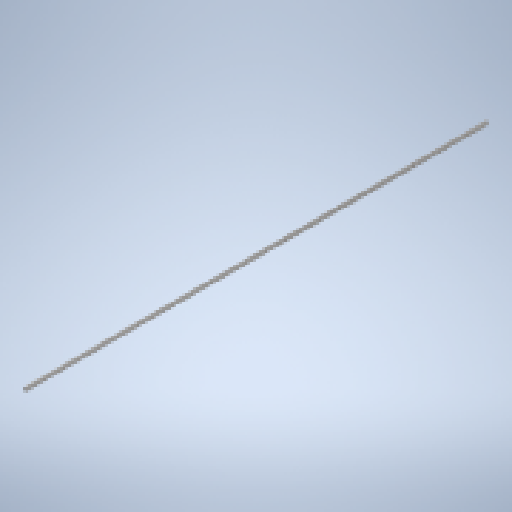
# Autodesk Inventor part: Guia Linear 490mm
Saved by Autodesk Inventor 2025.1 (Build 291241000, 241)
## iProperties
Created: 2020-11-03
Part Number: Guia Linear 490mm
Material: Aço, carbono
Document SubType Name: Modeling
Designer: Mateus
Density: 7.85 g/cm^3
Appearance: Semipolido
Author: Mateus
Autodesk Inventor part; units mm, degrees
ref_plane "YZ Plane" through (0, 0, 0) normal (1, 0, 0) x (0, 1, 0)
ref_plane "XZ Plane" through (0, 0, 0) normal (0, 1, 0) x (-1, 0, 0)
ref_plane "XY Plane" through (0, 0, 0) normal (0, 0, 1) x (1, 0, 0)
sketch "Esboço1" plane through (0, 0, 0) normal (0, 0, 1) x (1, 0, 0)
  circle A0 centre (0, 0) radius 4
  dimension "d0" = 8
  constraints: 1 centre point, 1 coincident
  measures "d0" diameter of A0
extrude "Extrusão1" add sketch "Esboço1" along normal blind 965
